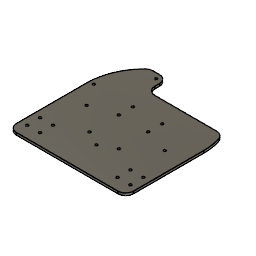
chasis v2 (Autodesk Fusion 360 design; units mm, degrees)
Autodesk Fusion 360 part; units mm, degrees
note: some values were not read from the file. Set by a fixed rule: which sketch regions a step uses.
sketch "Sketch1" plane through (0, 0, 0) normal (0, 0, 1) x (1, 0, 0)
  circle A0 centre (0, 0) radius 75
  line L0 (-75, 0) -> (75, 0)
  line L1 (75, 0) -> (75, -100)
  line L2 (75, -100) -> (-75, -100)
  line L3 (-75, -100) -> (-75, 0)
  circle A1 centre (49.5, -68.5) radius 1.55
  circle A2 centre (66, -85) radius 1.55
  circle A3 centre (66, -68.5) radius 1.55
  circle A4 centre (49.5, -85) radius 1.55
  circle A5 centre (-66, -68.5) radius 1.55
  circle A6 centre (-66, -85) radius 1.55
  circle A7 centre (-49.5, -68.5) radius 1.55
  circle A8 centre (-49.5, -85) radius 1.55
  line L4 (-50, 55.9017) -> (50, 55.9017)
  circle A9 centre (-18.75, -52.5) radius 1.55
  circle A10 centre (18.75, -52.5) radius 1.55
  circle A11 centre (18.75, -15) radius 1.55
  circle A12 centre (-18.75, -15) radius 1.55
  line L5 (-69, 49) -> (-35, 49)
  line L6 (-35, 49) -> (-35, 3)
  line L7 (-35, 3) -> (-69, 3)
  line L8 (-69, 3) -> (-69, 49)
  circle A13 centre (-69, 3) radius 1.5
  circle A14 centre (-35, 49) radius 1.5
  circle A15 centre (-35, 49) radius 3
  circle A16 centre (-69, 3) radius 3
  line L9 (-27.5, 69.7764) -> (-27.5, 29.7764)
  line L10 (-27.5, 29.7764) -> (68.8358, 29.7764)
  circle A17 centre (-18.75, 3) radius 1.5
  circle A18 centre (18.75, 3) radius 1.5
  circle A19 centre (-50, -25) radius 1.5
  circle A20 centre (50, -25) radius 1.5
  circle A21 centre (0, -62.5) radius 1.5
  dimension "d1" = 150
  dimension "d2" = 150
  dimension "d3" = 100
  dimension "d4" = 3.1
  dimension "d5" = 3.1
  dimension "d6" = 3.1
  dimension "d7" = 3.1
  dimension "d8" = 3.1
  dimension "d9" = 3.1
  dimension "d10" = 3.1
  dimension "d11" = 3.1
  dimension "d12" = 16.5
  dimension "d14" = 16.5
  dimension "d15" = 16.5
  dimension "d16" = 16.5
  dimension "d17" = 16.5
  dimension "d18" = 16.5
  dimension "d20" = 16.5
  dimension "d21" = 16.5
  dimension "d22" = 9
  dimension "d23" = 9
  dimension "d24" = 15
  dimension "d25" = 15
  dimension "d26" = 100
  dimension "d27" = 3.1
  dimension "d28" = 3.1
  dimension "d29" = 3.1
  dimension "d30" = 3.1
  dimension "d36" = 37.5
  dimension "d37" = 37.5
  dimension "d38" = 37.5
  dimension "d39" = 37.5
  dimension "d46" = 15
  dimension "d47" = 18.75
  dimension "d55" = 34
  dimension "d56" = 46
  dimension "d57" = 3
  dimension "d58" = 40
  dimension "d59" = 3
  dimension "d60" = 3
  dimension "d73" = 6
  dimension "d74" = 6
  dimension "d86" = 40
  dimension "d87" = 7.5
  dimension "d88" = 3
  dimension "d89" = 3
  dimension "d90" = 37.5
  dimension "d91" = 18.75
  dimension "d92" = 3
  dimension "d95" = 3
  dimension "d96" = 3
  dimension "d97" = 100
  dimension "d98" = 50
  dimension "d99" = 25
  dimension "d100" = 3
  dimension "d101" = 18.75
  dimension "d102" = 10
  constraint coincident A0.centre origin
  constraint horizontal L0
  constraint vertical L1
  constraint horizontal L2
  constraint vertical L3
  constraint midpoint A0.centre L0
  constraint vertical A5.centre A6.centre
  constraint vertical A2.centre A3.centre
  constraint horizontal A1.centre A3.centre
  constraint horizontal A5.centre A7.centre
  constraint coincident A0 L4.start
  constraint coincident A0 L4.end
  constraint horizontal L4
  constraint horizontal A11.centre A12.centre
  constraint vertical A10.centre A11.centre
  constraint horizontal L5
  constraint vertical L6
  constraint horizontal L7
  constraint vertical L8
  constraint coincident L7.end L8.start
  constraint coincident L5.end L6.start
  constraint concentric A14 A15
  constraint concentric A13 A16
  constraint coincident A0 L9.start
  constraint perpendicular L4 L9
  constraint coincident A0 L10.end
  constraint perpendicular L9 L10
  constraint horizontal A17.centre A18.centre
  constraint horizontal A19.centre A20.centre
  measures "d1" diameter of A0
  measures "d2" distance of L0.start L0.end
  measures "d3" distance of L0.start L2.end
  measures "d4" diameter of A1
  measures "d5" diameter of A2
  measures "d6" diameter of A3
  measures "d7" diameter of A4
  measures "d8" diameter of A5
  measures "d9" diameter of A6
  measures "d10" diameter of A7
  measures "d11" diameter of A8
  measures "d12" horizontal distance of A5.centre A7.centre
  measures "d14" vertical distance of A5.centre A6.centre
  measures "d15" horizontal distance of A6.centre A8.centre
  measures "d16" vertical distance of A7.centre A8.centre
  measures "d17" horizontal distance of A1.centre A3.centre
  measures "d18" vertical distance of A1.centre A4.centre
  measures "d20" horizontal distance of A2.centre A4.centre
  measures "d21" vertical distance of A2.centre A3.centre
  measures "d22" distance of L1 A2.centre
  measures "d23" distance of L3 A6.centre
  measures "d24" distance of L2 A6.centre
  measures "d25" distance of L2 A2.centre
  measures "d26" distance of L4.start L4.end
  measures "d27" diameter of A9
  measures "d28" diameter of A10
  measures "d29" diameter of A11
  measures "d30" diameter of A12
  measures "d36" vertical distance of A9.centre A12.centre
  measures "d37" horizontal distance of A9.centre A10.centre
  measures "d38" vertical distance of A10.centre A11.centre
  measures "d39" horizontal distance of A11.centre A12.centre
  measures "d46" distance of L0 A12.centre
  measures "d47" horizontal distance of A0.centre A12.centre
  measures "d55" distance of L5.start L5.end
  measures "d56" distance of L5.start L7.end
  measures "d57" distance of L0 L7
  measures "d58" horizontal distance of L0.start L5.end
  measures "d59" diameter of A13
  measures "d60" diameter of A14
  measures "d73" diameter of A15
  measures "d74" diameter of A16
  measures "d86" distance of L9.start L9.end
  measures "d87" distance of L6 L9
  measures "d88" diameter of A17
  measures "d89" diameter of A18
  measures "d90" distance of A17.centre A18.centre
  measures "d91" horizontal distance of A0.centre A17.centre
  measures "d92" vertical distance of A0.centre A18.centre
  measures "d95" diameter of A19
  measures "d96" diameter of A20
  measures "d97" horizontal distance of A19.centre A20.centre
  measures "d98" horizontal distance of A0.centre A20.centre
  measures "d99" vertical distance of A0.centre A19.centre
  measures "d100" diameter of A21
  measures "d101" horizontal distance of A10.centre A21.centre
  measures "d102" vertical distance of A10.centre A21.centre
extrude "Extrude7" add sketch "Sketch1" along normal blind 3 contours A0 L0 L4 L5 L6 L7 A15 A16 L9 L10 | A0 L1 L2 L3 | A0 L0 | A0 L0 L8 A16 | L7 L8 A13 A16 | A0 L5 L6 L7 L8 A15 A16 | L7 L8 A13 A16 | L5 L6 A14 A15 | L5 L6 A14 A15
fillet "Fillet6" radius 10 6 edges at (-27.5, 55.9017, 1.5) (75, -100, 1.5) (-75, -100, 1.5) (-50, 55.9017, 1.5) (68.8358, 29.7764, 1.5) (-27.5, 29.7764, 1.5)
